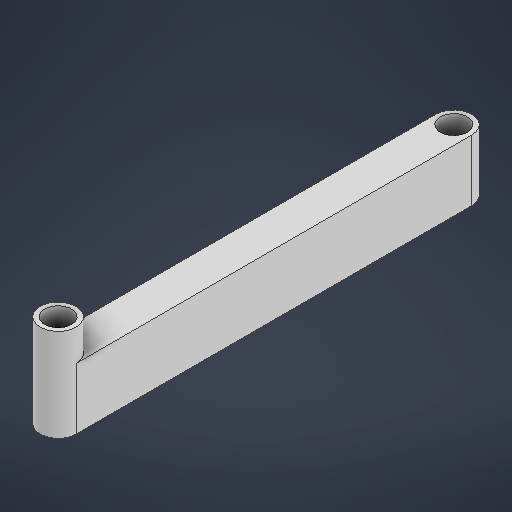
# Autodesk Inventor part: link_sub
Saved by Autodesk Inventor 2027 (Build 310192060, 192F)
## iProperties
Created: 2026-05-26
Part Number: link_sub
Material: Ogólny
Document SubType Name: Modeling
Designer: User
Density: 1 g/cm^3
Appearance: Domyślna
Author: User
Autodesk Inventor part; units mm, degrees
ref_plane "YZ Plane" through (0, 0, 0) normal (1, 0, 0) x (0, 1, 0)
ref_plane "XZ Plane" through (0, 0, 0) normal (0, 1, 0) x (-1, 0, 0)
ref_plane "XY Plane" through (0, 0, 0) normal (0, 0, 1) x (1, 0, 0)
sketch "Szkic1" plane through (0, 0, 0) normal (0, 1, 0) x (-1, 0, 0)
  circle A0 centre (0, 0) radius 1.5
  line L0 (-2, 2) -> (2, 2)
  line L1 (2, 2) -> (2, -2)
  line L2 (2, -2) -> (-2, -2)
  line L3 (-2, -2) -> (-2, 2)
  line L4 (-2, 2) -> (2, -2) construction
  line L5 (2, 2) -> (-2, -2) construction
  line L6 (0, 0) -> (0, -23)
  line L7 (0, 0) -> (23, 0) construction
  line L8 (2, 2) -> (-2, 2)
  line L9 (-2, 2) -> (-2, -22)
  line L10 (-2, -22) -> (2, -22)
  line L11 (2, -22) -> (2, 2)
  circle A1 centre (0, -44) radius 1.5
  line L12 (-2, -46) -> (2, -46)
  line L13 (2, -46) -> (2, -42)
  line L14 (2, -42) -> (-2, -42)
  line L15 (-2, -42) -> (-2, -46)
  line L16 (-2, -46) -> (2, -42) construction
  line L17 (2, -46) -> (-2, -42) construction
  line L18 (0, -44) -> (0, -23)
  line L19 (0, -44) -> (23, -44) construction
  line L20 (2, -46) -> (-2, -46)
  line L21 (-2, -46) -> (-2, -22)
  line L22 (2, -22) -> (2, -46)
  dimension "d0" = 3
  dimension "d1" = 4
  dimension "d2" = 4
  dimension "d3" = 23
  dimension "d4" = 90
  dimension "d5" = 4
  dimension "d6" = 24
  constraints: 46 end point, 8 symmetric about line, 4 parallel, 3 horizontal, 3 perpendicular, 2 centre point, 2 coincident, 2 midpoint, 1 vertical, 1 other
  measures "d0" diameter of A0
  measures "d1" distance of L1.end L2.end
  measures "d2" distance of L0.end L1.end
  measures "d3" distance of L6.start L6.end
  measures "d4" angle of L6 L7
  measures "d5" distance of L10.end L9.end
  measures "d6" distance of L9.end L8.end
extrude "Wyciągnięcie proste1" add sketch "Szkic1" along normal blind 6.8
fillet "Zaokrąglenie1" radius 2 4 edges at (-2, 3.4, 2) (2, 3.4, 2) (-2, 3.4, -46) (2, 3.4, -46)
sketch "Szkic2" plane through (0, 6.8, 0) normal (0, 1, 0) x (1, 0, 0)
  circle A0 centre (0, 0) radius 1.5 projected
  circle A1 centre (0, 0) radius 1.5
  circle A2 centre (0, 0) radius 2
  constraints: 2 centre point, 2 coincident
extrude "Wyciągnięcie proste2" add sketch "Szkic2" along normal blind 3.5
